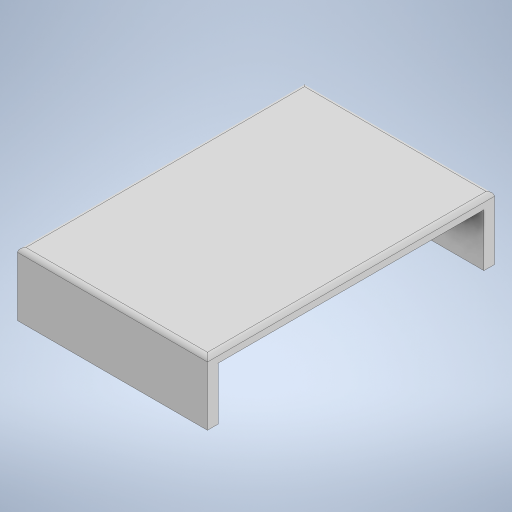
# Autodesk Inventor part: NavX_Box
Saved by Autodesk Inventor 2023 (Build 270158000, 158)
## iProperties
Created: 2023-02-01
Part Number: NavX_Box
Material: Generic
Document SubType Name: Modeling
Designer: linah
Density: 1 g/cm^3
Appearance: Default
Author: linah
Autodesk Inventor part; units mm, degrees
ref_plane "YZ Plane" through (0, 0, 0) normal (1, 0, 0) x (0, 1, 0)
ref_plane "XZ Plane" through (0, 0, 0) normal (0, 1, 0) x (-1, 0, 0)
ref_plane "XY Plane" through (0, 0, 0) normal (0, 0, 1) x (1, 0, 0)
sketch "Sketch1" plane through (0, 0, 0) normal (0, 1, 0) x (-1, 0, 0)
  line L0 (-57.15, -86.36) -> (57.15, -86.36)
  line L1 (57.15, -86.36) -> (57.15, 86.36)
  line L2 (57.15, 86.36) -> (-57.15, 86.36)
  line L3 (-57.15, 86.36) -> (-57.15, -86.36)
  line L4 (-57.15, -86.36) -> (57.15, 86.36) construction
  line L5 (57.15, -86.36) -> (-57.15, 86.36) construction
  point P0 (0, 0)
  dimension "d0" = 114.3
  dimension "d1" = 172.72
  constraints: 12 end point, 2 midpoint, 2 parallel, 1 horizontal, 1 perpendicular
  measures "d0" distance of L1.end L2.end
  measures "d1" distance of L0.end L1.end
extrude "Extrusion1" add sketch "Sketch1" along normal blind 38.1
sketch "Sketch2" plane through (57.15, 0, 86.36) normal (1, 0, 0) x (0, 0, -1)
  line L0 (6.35, 31.75) -> (166.37, 31.75)
  line L1 (166.37, 31.75) -> (166.37, 0)
  line L2 (166.37, 0) -> (6.35, 0)
  line L3 (6.35, 0) -> (6.35, 31.75)
  line L4 (0, 0) -> (172.72, 0) projected
  line L5 (172.72, 0) -> (172.72, 38.1) projected
  point P0 (86.36, 0)
  dimension "d4" = 160.02
  dimension "d5" = 31.75
  dimension "d6" = 0
  dimension "d7" = 6.35
  constraints: 8 end point, 2 parallel, 1 horizontal, 1 perpendicular
  measures "d4" distance of L1.end L2.end
  measures "d5" distance of L0.end L1.end
  measures "d6" distance between parallel lines of L4 L2
  measures "d7" distance between parallel lines of L5 L1
extrude "Extrusion2" cut sketch "Sketch2" against normal blind 127
fillet "Fillet1" radius 2.54 4 edges at (0, 38.1, 86.36) (0, 38.1, -86.36) (57.15, 38.1, 0) (-57.15, 38.1, 0)
body "Solid1"
